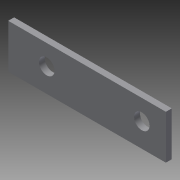
# Autodesk Inventor part: Bracket
Saved by Autodesk Inventor 2014 (Build 180170000, 170)
## iProperties
Created: 2014-01-06
Part Number: Bracket
Material: Generic
Document SubType Name: Modeling
Designer: Andrew Toennies
Density: 1 g/cm^3
Appearance: Default
Author: Andrew Toennies
Autodesk Inventor part; units mm, degrees
ref_plane "YZ Plane" through (0, 0, 0) normal (1, 0, 0) x (0, 1, 0)
ref_plane "XZ Plane" through (0, 0, 0) normal (0, 1, 0) x (-1, 0, 0)
ref_plane "XY Plane" through (0, 0, 0) normal (0, 0, 1) x (1, 0, 0)
sketch "Sketch1" plane through (0, 0, 0) normal (0, 0, 1) x (1, 0, 0)
  circle A0 centre (0, 0) radius 2.0828
  circle A1 centre (25.4, 0) radius 2.0828
  line L0 (25.4, 0) -> (0, 0) construction
  line L1 (-10.2931, 5.4128) -> (31.8265, 5.4128)
  line L2 (31.8265, 5.4128) -> (31.8265, -6.3559)
  line L3 (31.8265, -6.3559) -> (-10.2931, -6.3559)
  line L4 (-10.2931, -6.3559) -> (-10.2931, 5.4128)
  dimension "d0" = 4.1656
  dimension "d1" = 4.1656
  dimension "d2" = 25.4
  constraints: 10 end point, 2 centre point, 2 horizontal, 2 parallel, 1 coincident, 1 perpendicular
  measures "d0" diameter of A0
  measures "d1" diameter of A1
  measures "d2" distance of L0.end L0.start
extrude "Extrusion1" add sketch "Sketch1" along normal blind 1.5875
body "Solid1"
